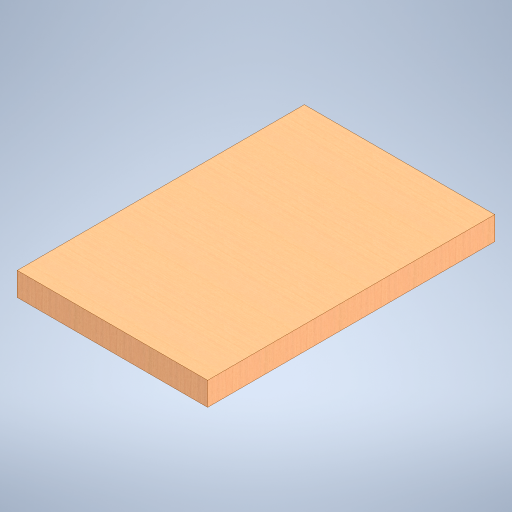
# Autodesk Inventor part: Caja Trigger DC
Saved by Autodesk Inventor 2024.2 (Build 282272000, 272)
## iProperties
Created: 2026-07-03
Part Number: Caja Trigger DC
Material: Wood (Cherry)
Document SubType Name: Modeling
Designer: ja.restrepo1
Density: 0.63 g/cm^3
Appearance: Cherry - Natural Low Gloss
Author: ja.restrepo1
Autodesk Inventor part; units mm, degrees
ref_plane "YZ Plane" through (0, 0, 0) normal (1, 0, 0) x (0, 1, 0)
ref_plane "XZ Plane" through (0, 0, 0) normal (0, 1, 0) x (-1, 0, 0)
ref_plane "XY Plane" through (0, 0, 0) normal (0, 0, 1) x (1, 0, 0)
sketch "Sketch1" plane through (0, 0, 0) normal (0, 1, 0) x (-1, 0, 0)
  line L0 (325, -490) -> (-325, -490)
  line L1 (-325, -490) -> (-325, 490)
  line L2 (-325, 490) -> (325, 490)
  line L3 (325, 490) -> (325, -490)
  point P0 (0, 0)
  point P1 (325, 0)
  point P2 (0, -490)
  dimension "d0" = 650
  dimension "d1" = 980
  constraints: 8 end point, 2 midpoint, 2 parallel, 1 horizontal, 1 horizontal alignment, 1 perpendicular, 1 vertical alignment
  measures "d0" distance of L1.end L2.end
  measures "d1" distance of L0.end L1.end
extrude "Caja MDF Trigger" add sketch "Sketch1" along normal blind 80
body "Solid1"
